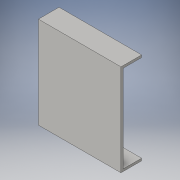
# Autodesk Inventor part: shaft chassis bracket
Saved by Autodesk Inventor 2016 SP2 (Build 200236200, 236)
## iProperties
Created: 2018-02-04
Part Number: shaft chassis bracket
Material: Generic
Document SubType Name: Modeling
Designer: CAD
Density: 1 g/cm^3
Appearance: Default
Author: CAD
Autodesk Inventor part; units mm, degrees
ref_plane "YZ Plane" through (0, 0, 0) normal (1, 0, 0) x (0, 1, 0)
ref_plane "XZ Plane" through (0, 0, 0) normal (0, 1, 0) x (-1, 0, 0)
ref_plane "XY Plane" through (0, 0, 0) normal (0, 0, 1) x (1, 0, 0)
sketch "Sketch1" plane through (0, 0, 0) normal (0, 0, 1) x (1, 0, 0)
  line L0 (0, 0) -> (0, 127)
  line L1 (0, 127) -> (114.3, 127)
  line L2 (114.3, 127) -> (114.3, 0)
  line L3 (114.3, 0) -> (0, 0)
  dimension "d0" = 127
  dimension "d1" = 114.3
  constraints: 8 end point, 2 perpendicular, 2 vertical
  measures "d0" distance of L0.start L0.end
  measures "d1" distance of L0.end L1.end
extrude "Extrusion1" add sketch "Sketch1" along normal blind 3.175
sketch "Sketch2" plane through (0, 0, 0) normal (0, 0, -1) x (-1, 0, 0)
  line L0 (-114.3, 0) -> (-114.3, 3.175)
  line L1 (-114.3, 0) -> (-114.3, 127) projected
  line L2 (-114.3, 3.175) -> (0, 3.175)
  line L3 (0, 127) -> (0, 0) projected
  line L4 (0, 3.175) -> (0, 0)
  line L5 (0, 0) -> (-114.3, 0)
  line L6 (0, 0) -> (-114.3, 0) projected
  line L7 (0, 63.5) -> (-19.05, 63.5)
  line L8 (-114.3, 127) -> (-114.3, 123.825)
  line L9 (-114.3, 127) -> (-114.3, 0)
  line L10 (-114.3, 123.825) -> (0, 123.825)
  line L11 (0, 0) -> (0, 127)
  line L12 (0, 123.825) -> (0, 127)
  line L13 (0, 127) -> (-114.3, 127)
  line L14 (0, 127) -> (-114.3, 127)
  dimension "d4" = 3.175
  constraints: 24 end point, 6 symmetric about line, 2 collinear, 2 point on line, 1 horizontal, 1 midpoint, 1 perpendicular
  measures "d4" distance of L0.start L0.end
extrude "Extrusion2" add sketch "Sketch2" along normal blind 25.4 contours L0 L2 L3 L5 | L1 L13 L3 L10
sketch "Sketch4" plane through (0, 0, 0) normal (0, 0, -1) x (-1, 0, 0)
  line L0 (0, 3.175) -> (0, 123.825) projected
  line L1 (-114.3, 0) -> (0, 0) projected
  point P0 (-57.15, 25.4)
  dimension "d16" = 57.15
  dimension "d17" = 25.4
  measures "d16" distance from line of L0 point (-57.15, 25.4)
  measures "d17" distance from line of L1 point (-57.15, 25.4)
hole "Hole1" at (57.15, 25.4, 0) direction (0, 0, 1) diameter 12.7 depth 1.5875
body "Solid1"
